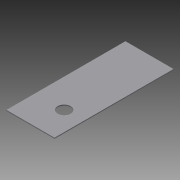
# Autodesk Inventor part: bearing plate
Saved by Autodesk Inventor 2015 (Build 190159000, 159)
## iProperties
Created: 2015-01-18
Part Number: bearing plate
Material: Generic
Document SubType Name: Modeling
Designer: chapale16
Density: 1 g/cm^3
Appearance: Default
Author: chapale16
Autodesk Inventor part; units mm, degrees
ref_plane "YZ Plane" through (0, 0, 0) normal (1, 0, 0) x (0, 1, 0)
ref_plane "XZ Plane" through (0, 0, 0) normal (0, 1, 0) x (-1, 0, 0)
ref_plane "XY Plane" through (0, 0, 0) normal (0, 0, 1) x (1, 0, 0)
sketch "Sketch1" plane through (0, 0, 0) normal (0, 1, 0) x (-1, 0, 0)
  line L0 (0, 0) -> (-149.225, 0)
  line L1 (-149.225, 0) -> (-149.225, -149.225)
  line L2 (-149.225, -149.225) -> (0, -149.225)
  line L3 (0, -149.225) -> (0, 0)
  circle A0 centre (-74.6125, -74.6125) radius 14.351
  dimension "d0" = 149.225
  dimension "d1" = 149.225
  dimension "d2" = 28.702
  constraints: 8 end point, 2 parallel, 1 centre point, 1 horizontal, 1 perpendicular
  measures "d0" distance of L2.end L1.end
  measures "d1" distance of L1.end L0.end
  measures "d2" diameter of A0
extrude "Extrusion1" add sketch "Sketch1" along normal blind 2.2098
sketch "Sketch5" plane through (0, 2.2098, 0) normal (0, 1, 0) x (1, 0, 0)
  circle A0 centre (74.6125, 74.6125) radius 14.351 projected
  line L0 (0, 0) -> (149.225, 0) projected
  line L1 (149.225, 0) -> (149.225, 149.225) projected
  line L2 (149.225, 149.225) -> (0, 149.225) projected
  line L3 (0, 149.225) -> (0, 0) projected
  line L4 (0, 0) -> (114.3, 0)
  line L5 (114.3, 0) -> (114.3, 257.2258)
  line L6 (114.3, 257.2258) -> (0, 257.2258)
  line L7 (0, 257.2258) -> (0, 0)
  dimension "d21" = 114.3
  dimension "d22" = 257.2258
  constraints: 8 end point, 2 parallel, 1 horizontal, 1 perpendicular
  measures "d21" distance of L6.end L5.end
  measures "d22" distance of L5.end L4.end
extrude "Extrusion6" add sketch "Sketch5" against normal blind 2.2098 contours L3 L2 L5 L0 | L7 L6 L5 L2
sketch "Sketch6" plane through (0, 2.2098, 0) normal (0, 1, 0) x (1, 0, 0)
  line L0 (114.3, 149.225) -> (149.225, 149.225)
  line L1 (149.225, 149.225) -> (149.225, 0)
  line L2 (149.225, 0) -> (114.3, 0)
  line L3 (114.3, 0) -> (114.3, 149.225)
  point P0 (0, 0)
  constraints: 8 end point, 2 parallel, 1 horizontal, 1 perpendicular
extrude "Extrusion7" cut sketch "Sketch6" against normal blind 2.2098
sketch "Sketch7" plane through (0, 2.2098, 0) normal (0, 1, 0) x (1, 0, 0)
  circle A0 centre (74.6125, 74.6125) radius 14.351 projected
  circle A1 centre (74.6125, 74.6125) radius 14.351
  point P0 (0, 0)
  constraints: 1 centre point, 1 coincident
extrude "Extrusion8" add sketch "Sketch7" against normal blind 2.2098
sketch "Sketch8" plane through (0, 2.2098, 0) normal (0, 1, 0) x (1, 0, 0)
  line L0 (0, 0) -> (114.3, 0) projected
  line L1 (16.637, 0) -> (97.663, 0)
  line L2 (16.637, 30.422) -> (16.637, 0)
  line L3 (16.637, 40.513) -> (57.15, 40.513)
  line L4 (57.15, 40.513) -> (57.15, 0)
  line L5 (57.15, 0) -> (16.637, 0)
  line L6 (16.637, 0) -> (16.637, 40.513)
  circle A0 centre (57.15, 40.513) radius 15.494
  dimension "d31" = 30.988
  constraints: 12 end point, 2 horizontal, 2 parallel, 1 centre point, 1 coincident, 1 midpoint, 1 perpendicular, 1 point on line
  measures "d31" diameter of A0
extrude "Extrusion9" cut sketch "Sketch8" against normal blind 2.2098 contours A0 L3 L4 | L4 L3 A0
sketch "Sketch9" plane through (0, 2.2098, 0) normal (0, 1, 0) x (1, 0, 0)
  circle A0 centre (57.15, 40.513) radius 15.494 projected
  line L0 (114.3, 0) -> (114.3, 257.2258) projected
  line L1 (114.3, 257.2258) -> (0, 257.2258) projected
  line L2 (0, 257.2258) -> (0, 0) projected
  line L3 (0, 0) -> (114.3, 0) projected
  line L4 (0, 0) -> (114.3, 0)
  line L5 (114.3, 0) -> (114.3, -25.4)
  line L6 (114.3, -25.4) -> (0, -25.4)
  line L7 (0, -25.4) -> (0, 0)
  line L8 (114.3, 257.2258) -> (114.3, 0) projected
  line L9 (0, 257.2258) -> (114.3, 257.2258)
  line L10 (114.3, 257.2258) -> (114.3, 231.8258)
  line L11 (114.3, 231.8258) -> (0, 231.8258)
  line L12 (0, 231.8258) -> (0, 257.2258)
  dimension "d34" = 25.4
  dimension "d35" = 25.4
  constraints: 16 end point, 4 parallel, 2 horizontal, 2 perpendicular, 1 point on line
  measures "d34" distance of L4.end L5.end
  measures "d35" distance of L9.end L10.end
extrude "Extrusion10" cut sketch "Sketch9" against normal blind 2.2098 contours L11 L2 L1 L0
extrude "Extrusion11" add sketch "Sketch9" against normal blind 2.2098 contours L5 L6 L7 L3
sketch "Sketch10" plane through (0, 2.2098, 0) normal (0, 1, 0) x (1, 0, 0)
  line L0 (0, -25.4) -> (25.4, -25.4)
  line L1 (25.4, -25.4) -> (25.4, 86.8868)
  line L2 (25.4, 86.8868) -> (0, 86.8868)
  line L3 (0, 86.8868) -> (0, -25.4)
  line L4 (114.3, -25.4) -> (114.3, 231.8258) projected
  line L5 (0, -25.4) -> (114.3, -25.4)
  line L6 (114.3, -25.4) -> (114.3, 0)
  line L7 (114.3, 0) -> (0, 0)
  line L8 (0, 0) -> (0, -25.4)
  line L9 (114.3, 231.8258) -> (0, 231.8258) projected
  line L10 (0, 231.8258) -> (0, -25.4) projected
  line L11 (0, -25.4) -> (114.3, -25.4) projected
  line L12 (114.3, -25.4) -> (114.3, 231.8258) projected
  circle A0 centre (57.15, 40.513) radius 15.494 projected
  circle A1 centre (57.15, 40.513) radius 15.494
  dimension "d40" = 25.4
  constraints: 16 end point, 4 parallel, 2 horizontal, 2 perpendicular, 1 centre point, 1 coincident, 1 concentric, 1 point on line
  measures "d40" distance of L2.end L1.end
extrude "Extrusion12" add sketch "Sketch10" against normal blind 2.2098 contours A0
sketch "Sketch11" plane through (0, 2.2098, 0) normal (0, 1, 0) x (1, 0, 0)
  line L0 (25.3965, 0) -> (68.5765, 0)
  line L1 (68.5765, 0) -> (68.5765, 43.18)
  line L2 (68.5765, 43.18) -> (25.3965, 43.18)
  line L3 (25.3965, 43.18) -> (25.3965, 0)
  circle A0 centre (68.5765, 43.18) radius 15.494
  point P0 (0, 0)
  dimension "d43" = 43.18
  dimension "d44" = 43.18
  dimension "d45" = 30.988
  constraints: 8 end point, 2 parallel, 1 centre point, 1 coincident, 1 horizontal, 1 perpendicular
  measures "d43" distance of L2.end L1.end
  measures "d44" distance of L1.end L0.end
  measures "d45" diameter of A0
extrude "Extrusion13" cut sketch "Sketch11" against normal blind 2.2098 contours A0 L2 L1 | L1 L2 A0
sketch "Sketch12" plane through (0, 2.2098, 0) normal (0, 1, 0) x (1, 0, 0)
  circle A0 centre (68.5765, 43.18) radius 15.494 projected
  line L0 (114.3, 231.8258) -> (0, 231.8258) projected
  line L1 (0, 231.8258) -> (0, -25.4) projected
  line L2 (0, -25.4) -> (114.3, -25.4) projected
  line L3 (114.3, -25.4) -> (114.3, 231.8258) projected
  line L4 (0, 231.8258) -> (114.3, 231.8258)
  line L5 (114.3, 231.8258) -> (114.3, 257.2258)
  line L6 (114.3, 257.2258) -> (0, 257.2258)
  line L7 (0, 257.2258) -> (0, 231.8258)
  point P0 (0, 0)
  dimension "d48" = 25.4
  constraints: 8 end point, 2 parallel, 1 horizontal, 1 perpendicular
  measures "d48" distance of L5.end L4.end
extrude "Extrusion14" add sketch "Sketch12" against normal blind 2.2098 contours L0 L7 L6 L5
body "Solid1"
